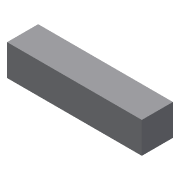
# Autodesk Inventor part: おもり1
Saved by Autodesk Inventor 2013 (Build 170138000, 138)
## iProperties
Created: 2014-02-06
Part Number: おもり1
Material: 一般
Document SubType Name: Modeling
Designer: victor
Density: 1 g/cm^3
Author: victor
Autodesk Inventor part; units mm, degrees
ref_plane "YZ Plane" through (0, 0, 0) normal (1, 0, 0) x (0, 1, 0)
ref_plane "XZ Plane" through (0, 0, 0) normal (0, 1, 0) x (-1, 0, 0)
ref_plane "XY Plane" through (0, 0, 0) normal (0, 0, 1) x (1, 0, 0)
sketch "スケッチ1" plane through (0, 0, 0) normal (0, 0, 1) x (1, 0, 0)
  line L0 (-35.2964, 5.4924) -> (29.7036, 5.4924)
  line L1 (29.7036, 5.4924) -> (29.7036, -9.5076)
  line L2 (29.7036, -9.5076) -> (-35.2964, -9.5076)
  line L3 (-35.2964, -9.5076) -> (-35.2964, 5.4924)
  point P0 (0, 0)
  dimension "d0" = 65
  dimension "d3" = 15
  constraints: 8 end point, 2 parallel, 1 horizontal, 1 perpendicular
  measures "d0" distance between parallel lines of L1 L3
  measures "d3" distance of L0.end L1.end
extrude "押し出し1" add sketch "スケッチ1" along normal blind 15
